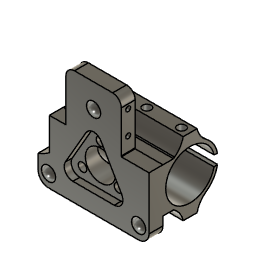
vacuum_pump_holder v3 (Autodesk Fusion 360 design; units mm, degrees)
Autodesk Fusion 360 part; units mm, degrees
sketch "Sketch1" plane through (0, 0, 0) normal (0, 1, 0) x (1, 0, 0)
  line L0 (-10.392305, 11.9) -> (10.392305, 11.9)
  arc A0 (-4.330127, -16.3) -> (4.330127, -16.3) centre (0, -13.8) ccw
  circle A1 centre (-25.980762, 15) radius 4.4
  circle A2 centre (0, -12) radius 2.475
  line L1 (0, 22.203919) -> (-7.3, 22.203919)
  line L2 (-16, -39.796081) -> (-16, -14.796081)
  line L3 (-11.951151, 11.9) -> (-10.392305, 11.9)
  line L4 (-32, 22.203919) -> (0, 22.203919)
  line L5 (32, 22.203919) -> (0, 22.203919)
  line L6 (5.10955, -14.95) -> (15.501855, 3.05)
  line L7 (-5.10955, -14.95) -> (-15.501855, 3.05)
  line L8 (0, -39.796081) -> (-16, -39.796081)
  line L9 (-32, -39.796081) -> (-32, 22.203919)
  arc A3 (-16, -14.796081) -> (-32, 7.874185) centre (-40.060655, -14.796081) ccw
  arc A4 (16.281278, 4.4) -> (11.951151, 11.9) centre (11.951151, 6.9) ccw
  circle A5 centre (0, 0) radius 8.75
  circle A6 centre (10.392305, 6) radius 2.475
  circle A7 centre (-10.392305, 6) radius 2.475
  line L10 (32, -39.796081) -> (32, 22.203919)
  line L11 (5.10955, -14.95) -> (4.330127, -16.3)
  line L12 (16, -39.796081) -> (16, -14.796081)
  line L13 (15.501855, 3.05) -> (16.281278, 4.4)
  arc A8 (32, 7.874185) -> (16, -14.796081) centre (40.060655, -14.796081) ccw
  line L14 (0, -39.796081) -> (16, -39.796081)
  arc A9 (-11.951151, 11.9) -> (-16.281278, 4.4) centre (-11.951151, 6.9) ccw
  circle A10 centre (25.980762, 15) radius 4.4
  line L15 (11.951151, 11.9) -> (10.392305, 11.9)
  line L16 (-5.10955, -14.95) -> (-4.330127, -16.3)
  line L17 (-15.501855, 3.05) -> (-16.281278, 4.4)
  circle A11 centre (0, -30) radius 1.6
  line L18 (-32, -39.796081) -> (-16, -39.796081)
  line L19 (16, -39.796081) -> (32, -39.796081)
  line L20 (-32, 22.203919) -> (-32, -1.546081)
  line L21 (-32, -1.546081) -> (-32, -13.796081)
  line L22 (32, 22.203919) -> (32, -1.546081)
  line L23 (32, -1.546081) -> (32, -15.546081)
  line L24 (0, 22.203919) -> (-12, 22.203919)
  line L25 (0, 22.203919) -> (12, 22.203919)
  line L26 (-12, 22.203919) -> (-12, 17.203919)
  circle A12 centre (12, 16.203919) radius 1.45
  circle A13 centre (12, -28.796081) radius 1.45
  line L27 (32, -39.796081) -> (32, -25.296081)
  arc A14 (32, -25.296081) -> (16, -39.796081) centre (30.570312, -39.796081) ccw
  line L28 (0, 0) -> (0, 22.203919)
  arc A15 (-16, -39.796081) -> (-32, -25.296081) centre (-30.570312, -39.796081) ccw
  circle A16 centre (-12, 16.203919) radius 1.45
  circle A17 centre (-12, -28.796081) radius 1.45
  line L29 (-32, -39.796081) -> (-32, -14.326081)
  arc A18 (-16, -39.796081) -> (-32, -14.326081) centre (-40.951887, -37.710087) ccw
  line L30 (-32, -14.326081) -> (-25.5, -14.326081)
  line L31 (-25.5, -14.326081) -> (-25.5, 4.358617)
  arc A19 (32, -14.326081) -> (16, -39.796081) centre (40.951887, -37.710087) ccw
  line L32 (-32, -14.326081) -> (-16.004591, -14.326081)
  line L33 (32, -14.326081) -> (16.004591, -14.326081)
  circle A20 centre (-25.980762, 15) radius 2.8
  circle A21 centre (25.980762, 15) radius 2.8
  circle A22 centre (0, -30) radius 2.8
  circle A23 centre (25.980762, 15) radius 1.75
  point P0 (-25.980762, 15)
  point P1 (25.980762, 15)
  dimension "d1" = 17.5
  dimension "d2" = 12
  dimension "d3" = 4.95
  dimension "d4" = 4.95
  dimension "d5" = 4.95
  dimension "d6" = 5.9
  dimension "d7" = 5.9
  dimension "d8" = 5
  dimension "d9" = 3.2
  dimension "d10" = 8.8
  dimension "d11" = 8.8
  dimension "d12" = 16
  dimension "d13" = 16
  dimension "d14" = 62
  dimension "d15" = 25
  dimension "d78" = 23.75
  dimension "d80" = 23.75
  dimension "d81" = 14
  dimension "d90" = 12
  dimension "d91" = 12
  dimension "d96" = 5
  dimension "d97" = 6
  dimension "d99" = 2.9
  dimension "d136" = 45
  dimension "d137" = 2.9
  dimension "d141" = 14.5
  dimension "d218" = 25.47
  dimension "d219" = 6.5
  dimension "d234" = 5.6
  dimension "d235" = 5.6
  dimension "d236" = 5.6
  dimension "d239" = 3.5
  constraint tangent A0 L11
  constraint tangent A0 L16
  constraint tangent A4 L13
  constraint tangent A4 L15
  constraint equal A0 A4
  constraint tangent L3 A9
  constraint tangent A9 L17
  constraint equal A0 A9
  constraint perpendicular L5 L10
  constraint tangent L12 A8
  constraint parallel L1 L4
  constraint perpendicular L2 L18
  constraint perpendicular L10 L19
  constraint perpendicular L4 L20
  constraint parallel L9 L21
  constraint perpendicular L5 L22
  constraint parallel L10 L23
  constraint parallel L4 L24
  constraint parallel L5 L25
  constraint perpendicular L4 L26
  constraint perpendicular L19 L27
  constraint tangent L12 A14
  constraint coincident A5.centre L28.start
  constraint perpendicular L4 L28
  constraint symmetric A14 L28 A15
  constraint symmetric A12 L28 A16
  constraint symmetric A13 L28 A17
  constraint perpendicular L18 L29
  constraint perpendicular L9 L30
  constraint perpendicular L30 L31
  constraint symmetric L28 A18 A19
  constraint perpendicular L2 L32
  constraint concentric A1 A20
  constraint concentric A10 A21
  constraint concentric A11 A22
  measures "d1" diameter of A5
  measures "d3" diameter of A2
  measures "d4" diameter of A6
  measures "d5" diameter of A7
  measures "d8" radius of A0
  measures "d9" diameter of A11
  measures "d10" diameter of A1
  measures "d11" diameter of A10
  measures "d99" diameter of A12
  measures "d137" diameter of A13
  measures "d234" diameter of A20
  measures "d235" diameter of A21
  measures "d236" diameter of A22
  measures "d239" diameter of A23
sketch "bottom" plane through (0, 0, 39.796081) normal (0, 0, 1) x (-1, 0, 0)
  line L0 (32, 0) -> (-32, 0)
  line L1 (-32, 0) -> (-32, -10)
  line L2 (-32, -10) -> (32, -10)
  line L3 (32, -10) -> (32, 0)
  line L4 (32, 0) -> (32, -19.73)
  line L5 (-32, 0) -> (-32, -19.73)
  line L6 (0, 0) -> (0, -19.73)
  circle A0 centre (0, -19.73) radius 14
  circle A1 centre (0, -19.73) radius 12.25
  line L7 (0, -19.73) -> (21.8, -19.73)
  line L8 (21.8, -19.73) -> (21.8, -22.73)
  line L9 (21.8, -19.73) -> (21.8, -16.73)
  line L10 (21.8, -16.73) -> (13.674794, -16.73)
  line L11 (21.8, -22.73) -> (13.674794, -22.73)
  line L12 (0, -30) -> (12, -30)
  line L13 (0, -30) -> (-12, -30)
  arc A2 (-12, -30) -> (12, -30) centre (0, -20.125001) ccw
  line L14 (32, -19.73) -> (12, -30)
  line L15 (-12, -30) -> (-32, -19.73)
  dimension "d22" = 19.73
  dimension "d23" = 19.73
  dimension "d29" = 19.73
  dimension "d30" = 28
  dimension "d31" = 24.5
  dimension "d32" = 21.8
  dimension "d33" = 3
  dimension "d34" = 3
  dimension "d35" = 12
  constraint coincident L0.start L3.end
  constraint perpendicular L0 L4
  constraint coincident L0.end L1.start
  constraint perpendicular L0 L5
  constraint coincident L6.start origin
  constraint perpendicular L0 L6
  constraint coincident L6.end A0.centre
  constraint concentric A0 A1
  constraint perpendicular L6 L7
  constraint perpendicular L7 L8
  constraint perpendicular L7 L9
  constraint perpendicular L9 L10
  constraint perpendicular L8 L11
  constraint horizontal L12
  constraint parallel L12 L13
  measures "d22" distance of L0.start L4.end
  measures "d23" distance of L0.end L5.end
  measures "d29" distance of L6.start L6.end
  measures "d30" diameter of A0
  measures "d31" diameter of A1
  measures "d32" distance of L6.end L7.end
  measures "d33" distance of L7.end L8.end
  measures "d34" distance of L7.end L9.end
  measures "d35" distance of L12.start L13.end
extrude "Extrude4" add sketch "Sketch1" along normal blind 39.46 contours L0 A0 L3 L6 L7 A4 L11 L13 A9 L15 L16 L17 | A1 | A2 | L1 L2 L4 L5 L8 L9 A3 L10 L12 A8 L14 L20 L22 L24 L25 A18 A19 | L10 A8 L22 L23 L33 | L9 A3 L20 L21 L30 L31 L32 | L12 A8 A19 L33 | A3 L31 L32 | L10 L12 L23 A14 A19 | L2 A3 A18 L30 L32 | L12 A19 | L2 L9 A15 L29 A18 | L10 L19 L27 A14 | L9 L18 A15 L29 | L2 A18 | A5 | A6 | A7 | A10 | A11 | A12 | A13 | A16 | A17 | A20 | A21 | A22 | A23 picked at (-4.711137, 10.569969) picked at (-22.140901, 14.642299) picked at (-0.18358, -11.195684) picked at (-10.740589, -19.482072) picked at (27.37273, -6.932301) picked at (-27.666667, -3.837848) picked at (20.054611, -19.162446) picked at (-19.256218, -13.297778) picked at (28.224316, -19.587338) picked at (-21.577044, -16.380874) picked at (15.974211, -37.478071) picked at (-30.939878, -18.476301) picked at (21.380237, -39.122729) picked at (-21.380237, -39.122729) picked at (-15.974211, -37.942103) picked at (-0.424451, 2.741984) picked at (10.956125, 6.501084) picked at (-10.123158, 6.626633) picked at (29.820623, 14.642299) picked at (-0.142372, -29.637241) picked at (12.435468, 15.994209) picked at (12.46186, -28.938546) picked at (-11.895495, 15.822215) picked at (-11.53814, -28.938546) picked at (-25.639777, 14.04895) picked at (28.413822, 14.773953) picked at (2.383619, -30.218595) picked at (27.031686, 14.71542)
sketch "side2" plane through (32, 0, 0) normal (1, 0, 0) x (0, 1, 0)
  line L0 (0, 39.796081) -> (0, -22.203919)
  line L1 (0, -22.203919) -> (39.46, -22.203919)
  line L2 (39.46, -22.203919) -> (39.46, 39.796081)
  line L3 (39.46, 39.796081) -> (0, 39.796081)
  line L4 (19.73, -22.203919) -> (5.73, -22.203919)
  circle A0 centre (19.73, 1.546081) radius 14.1
  circle A1 centre (19.73, 1.546081) radius 16
  line L5 (19.73, 1.546081) -> (19.73, 4.546081)
  line L6 (19.73, 4.546081) -> (43.73, 4.546081)
  line L7 (43.73, 4.546081) -> (43.73, -1.453919)
  line L8 (43.73, -1.453919) -> (35.446234, -1.453919)
  line L9 (19.73, 1.546081) -> (43.73, 1.546081)
  line L10 (0, -22.203919) -> (4, -22.203919)
  line L11 (4, -22.203919) -> (4, 39.796081)
  line L12 (4, -22.203919) -> (4, -17.203919)
  line L13 (39.46, 1.546081) -> (39.46, -4.453919)
  line L14 (39.46, 1.546081) -> (39.46, 7.546081)
  line L15 (43.73, 4.546081) -> (39.46, 7.546081)
  line L16 (39.46, 7.546081) -> (29.357219, 14.325621)
  line L17 (39.46, -4.453919) -> (29.357219, -11.23346)
  line L18 (43.73, -1.453919) -> (39.46, -4.453919)
  line L19 (39.46, 25.296081) -> (4, 25.296081)
  line L20 (29.357219, 14.325621) -> (29.357219, 25.296081)
  line L21 (29.357219, -11.23346) -> (29.357219, -22.203919)
  line L22 (19.73, 17.546081) -> (19.73, 22.546081)
  line L23 (19.73, 22.546081) -> (29.357219, 22.546081)
  line L24 (19.73, 22.546081) -> (23.73, 22.546081)
  line L25 (19.73, 22.546081) -> (4, 22.546081)
  arc A2 (23.73, 22.546081) -> (29.357219, 14.325621) centre (36.849635, 25.49072) ccw
  arc A3 (4, 25.296081) -> (19.73, 22.546081) centre (20.714595, 74.540765) ccw
  line L26 (19.73, -19.453919) -> (23.73, -19.453919)
  arc A4 (29.357219, -11.23346) -> (23.73, -19.453919) centre (36.849635, -22.398558) ccw
  arc A5 (19.73, -19.453919) -> (4, -22.203919) centre (20.714595, -71.448604) ccw
  arc A6 (10.102781, 14.325621) -> (15.73, 22.546081) centre (2.610365, 25.49072) ccw
  arc A7 (4, 22.546081) -> (10.102781, 14.325621) centre (41.738131, 44.186915) ccw
  arc A8 (15.73, -19.453919) -> (10.102781, -11.23346) centre (2.610365, -22.398558) ccw
  line L27 (15.73, -19.453919) -> (23.73, -19.453919)
  line L28 (10.102781, 14.325621) -> (4, 14.325621)
  line L29 (10.102781, -11.23346) -> (4, -11.23346)
  line L30 (35.446234, -1.453919) -> (33.507155, -1.453919)
  line L31 (33.507155, 4.546081) -> (40.904794, 4.546081)
  line L32 (40.904794, 1.546081) -> (40.904794, -0.953919)
  line L33 (40.904794, 1.546081) -> (40.904794, 4.046081)
  arc A9 (33.507155, 4.546081) -> (40.904794, 4.046081) centre (40.110525, 47.269716) ccw
  arc A10 (40.904794, -0.953919) -> (33.507155, -1.453919) centre (40.110525, -44.177555) ccw
  line L34 (0, 39.796081) -> (-4, 39.796081)
  dimension "d50" = 19.73
  dimension "d53" = 14
  dimension "d60" = 28.2
  dimension "d102" = 32
  dimension "d105" = 3
  dimension "d107" = 24
  dimension "d108" = 6
  dimension "d114" = 4
  dimension "d115" = 5
  dimension "d118" = 6
  dimension "d119" = 6
  dimension "d165" = 5
  dimension "d166" = 4
  dimension "d171" = 2.5
  dimension "d172" = 2.5
  dimension "d251" = 4
  constraint concentric A0 A1
  constraint vertical L5
  constraint perpendicular L2 L6
  constraint perpendicular L6 L7
  constraint perpendicular L5 L8
  constraint perpendicular L0 L10
  constraint perpendicular L3 L11
  constraint perpendicular L10 L12
  constraint perpendicular L8 L13
  constraint perpendicular L6 L14
  constraint perpendicular L11 L19
  constraint perpendicular L19 L20
  constraint perpendicular L1 L21
  constraint perpendicular L19 L22
  constraint perpendicular L20 L23
  constraint perpendicular L22 L24
  constraint perpendicular L11 L25
  constraint tangent L16 A2
  constraint symmetric L9 A2 A4
  constraint symmetric L9 A3 A5
  constraint symmetric L22 A2 A6
  constraint symmetric L9 A6 A8
  constraint perpendicular L11 L28
  constraint perpendicular L11 L29
  constraint parallel L8 L30
  constraint perpendicular L14 L31
  constraint perpendicular L9 L32
  constraint perpendicular L9 L33
  constraint symmetric L9 A9 A10
  constraint perpendicular L0 L34
  measures "d60" diameter of A0
  measures "d102" diameter of A1
sketch "top" plane through (0, 39.46, 0) normal (0, 1, 0) x (-1, 0, 0)
  line L0 (32, 39.796081) -> (-32, 39.796081)
  line L1 (-32, 39.796081) -> (-32, -22.203919)
  line L2 (-32, -22.203919) -> (32, -22.203919)
  line L3 (32, -22.203919) -> (32, 39.796081)
  line L4 (-32, -22.203919) -> (-32, -12.203919)
  line L5 (-32, -12.203919) -> (-4.5, -12.203919)
  line L6 (-4.5, -12.203919) -> (-4.5, 15.796081)
  line L7 (-4.5, 15.796081) -> (-32, 15.796081)
  line L8 (-4.5, -12.203919) -> (-4.5, 1.796081)
  line L9 (-32, -12.203919) -> (-32, 1.796081)
  line L10 (-32, 1.796081) -> (-13.1, 1.796081)
  circle A0 centre (-13.1, 1.796081) radius 3
  line L11 (-32, 1.796081) -> (25.5, 1.796081)
  line L12 (25.5, 1.796081) -> (25.5, 14.046081)
  line L13 (25.5, 14.046081) -> (-4.5, 14.046081)
  line L14 (25.5, -10.453919) -> (-4.5, -10.453919)
  line L15 (25.5, 1.796081) -> (25.5, -10.453919)
  line L16 (32, 39.796081) -> (-32, 39.796081)
  line L17 (0, -22.203919) -> (-12, -22.203919)
  line L18 (0, -22.203919) -> (12, -22.203919)
  line L19 (-12, -22.203919) -> (-12, -16.203919)
  circle A1 centre (-12, -16.203919) radius 2.75
  line L20 (12, -22.203919) -> (12, -16.203919)
  circle A2 centre (12, -16.203919) radius 2.75
  circle A3 centre (-12, 28.796081) radius 2.75
  line L21 (0, 39.796081) -> (0, -22.203919)
  circle A4 centre (12, 28.796081) radius 2.75
  dimension "d61" = 10
  dimension "d62" = 27.5
  dimension "d63" = 28
  dimension "d64" = 14
  dimension "d65" = 18.9
  dimension "d66" = 6
  dimension "d67" = 57.5
  dimension "d68" = 12.25
  dimension "d126" = 12
  dimension "d127" = 12
  dimension "d128" = 6
  dimension "d129" = 5.5
  dimension "d130" = 6
  dimension "d131" = 5.5
  dimension "d139" = 45
  dimension "d140" = 5.5
  constraint perpendicular L2 L4
  constraint perpendicular L4 L5
  constraint perpendicular L5 L6
  constraint perpendicular L1 L7
  constraint perpendicular L5 L9
  constraint perpendicular L9 L10
  constraint perpendicular L9 L11
  constraint perpendicular L11 L12
  constraint perpendicular L6 L13
  constraint parallel L2 L17
  constraint parallel L2 L18
  constraint perpendicular L17 L19
  constraint perpendicular L18 L20
  constraint symmetric A3 L21 A4
  measures "d66" diameter of A0
  measures "d129" diameter of A1
  measures "d131" diameter of A2
  measures "d140" diameter of A3
sketch "side1" plane through (-32, 0, 0) normal (-1, 0, 0) x (0, -1, 0)
  line L0 (0, -22.203919) -> (0, 39.796081)
  line L1 (0, 39.796081) -> (-39.46, 39.796081)
  line L2 (-39.46, 39.796081) -> (-39.46, -22.203919)
  line L3 (-39.46, -22.203919) -> (0, -22.203919)
  line L4 (0, -22.203919) -> (-19.73, -22.203919)
  line L5 (-19.73, -22.203919) -> (-19.73, 1.546081)
  circle A0 centre (-19.73, 1.546081) radius 12.65
  line L6 (0, -22.203919) -> (-4, -22.203919)
  line L7 (-4, -22.203919) -> (-4, 39.796081)
  line L8 (-41.73, 4.546081) -> (-41.73, -1.453919)
  circle A1 centre (-19.73, 1.546081) radius 14.25
  line L9 (-4, -22.203919) -> (-4, -17.203919)
  arc A2 (-41.73, 4.546081) -> (-29.866601, 11.56166) centre (-49.126004, 30.591122) ccw
  arc A3 (-29.866601, -8.469498) -> (-41.73, -1.453919) centre (-49.126004, -27.498961) ccw
  arc A4 (-4, -22.203919) -> (-19.73, -12.703919) centre (-19.496567, -30.090188) ccw
  arc A5 (-19.73, 15.796081) -> (-4, 25.296081) centre (-19.496567, 33.18235) ccw
  circle A6 centre (-19.73, 1.546081) radius 3.25
  circle A7 centre (-19.73, 1.546081) radius 10
  circle A8 centre (-19.73, 1.546081) radius 8.15
  circle A9 centre (-19.73, 1.546081) radius 13
  circle A10 centre (-19.73, 1.546081) radius 7
  line L10 (-19.73, 4.796081) -> (-31.955383, 4.796081)
  line L11 (-19.73, -1.703919) -> (-31.955383, -1.703919)
  line L12 (-19.73, 4.796081) -> (-7.504617, 4.796081)
  line L13 (-19.73, -1.703919) -> (-7.504617, -1.703919)
  dimension "d71" = 19.73
  dimension "d72" = 23.75
  dimension "d73" = 25.3
  dimension "d82" = 4
  dimension "d111" = 6
  dimension "d112" = 28.5
  dimension "d113" = 5
  dimension "d179" = 6.5
  dimension "d180" = 20
  dimension "d181" = 16.3
  dimension "d182" = 26
  dimension "d190" = 14
  constraint perpendicular L0 L4
  constraint perpendicular L4 L5
  constraint perpendicular L0 L6
  constraint perpendicular L1 L7
  constraint concentric A0 A1
  constraint perpendicular L4 L9
  constraint tangent A1 A2
  constraint concentric A0 A6
  constraint concentric A1 A7
  constraint concentric A6 A8
  constraint concentric A7 A9
  constraint concentric A8 A10
  constraint tangent A6 L10
  constraint horizontal L10
  constraint tangent A6 L11
  constraint parallel L11 L12
  constraint parallel L12 L13
  measures "d73" diameter of A0
  measures "d112" diameter of A1
  measures "d179" diameter of A6
  measures "d180" diameter of A7
  measures "d181" diameter of A8
  measures "d182" diameter of A9
  measures "d190" diameter of A10
sketch "high" plane through (0, 0, 39.796081) normal (0, 0, 1) x (-1, 0, 0)
  line L0 (32, 0) -> (-32, 0)
  line L1 (-32, 0) -> (-32, -39.46)
  line L2 (-32, -39.46) -> (32, -39.46)
  line L3 (32, -39.46) -> (32, 0)
  line L4 (-32, 0) -> (-32, -19.73)
  line L5 (-32, -19.73) -> (-27, -19.73)
  circle A0 centre (-27, -19.73) radius 2.45
  line L6 (-4.5, -5.73) -> (-32, -5.73)
  line L7 (-4.5, -33.73) -> (-4.5, -5.73)
  line L8 (-32, -33.73) -> (-4.5, -33.73)
  line L9 (25.5, -31.98) -> (-4.5, -31.98)
  line L10 (25.5, -19.73) -> (25.5, -31.98)
  line L11 (25.5, -19.73) -> (25.5, -7.48)
  line L12 (25.5, -7.48) -> (-4.5, -7.48)
  line L13 (-32, -39.46) -> (25.5, -39.46)
  circle A1 centre (-7, -19.73) radius 2.45
  circle A2 centre (7, -19.73) radius 2.45
  line L14 (16, -19.73) -> (7, -19.73)
  line L15 (16, -19.73) -> (7, -19.73)
  line L16 (16, -19.73) -> (-16, -19.73)
  point P0 (-32, -19.73)
  point P1 (25.5, -19.73)
  point P2 (-7, -19.73)
  point P3 (7, -19.73)
  dimension "d158" = 5
  dimension "d159" = 4.9
  dimension "d199" = 27.5
  dimension "d200" = 28
  dimension "d201" = 12.25
  dimension "d202" = 57.5
  dimension "d203" = 19.73
  dimension "d215" = 4.9
  dimension "d217" = 4.9
  dimension "d244" = 9
  constraint coincident L0.end L1.start
  constraint midpoint L1 P0
  constraint perpendicular L4 L5
  constraint coincident L5.end A0.centre
  constraint perpendicular L7 L8
  constraint coincident L12.end L7
  constraint perpendicular L7 L12
  constraint coincident L1.end L2.start
  constraint perpendicular L1 L13
  constraint coincident P0 L4.end
  constraint parallel L14 L15
  constraint coincident P3 A2.centre
  constraint parallel L14 L16
  measures "d158" distance of P0 L5.end
  measures "d159" diameter of A0
  measures "d199" distance of L7.start L8.start
  measures "d200" distance of L7.start L6.start
  measures "d201" distance of L11.end P1
  measures "d202" distance of L1.end L13.end
  measures "d203" distance of L13.end P1
  measures "d215" diameter of A1
  measures "d217" diameter of A2
  measures "d244" distance of L14.start P3
sketch "low" plane through (0, 0, -22.203919) normal (0, 0, -1) x (1, 0, 0)
  line L0 (32, 0) -> (-32, 0)
  line L1 (-32, 0) -> (-32, -39.46)
  line L2 (-32, -39.46) -> (32, -39.46)
  line L3 (32, -39.46) -> (32, 0)
  line L4 (32, -39.46) -> (32, -19.73)
  line L5 (32, -19.73) -> (27, -19.73)
  circle A0 centre (27, -19.73) radius 1.425
  line L6 (32, -19.73) -> (12, -19.73)
  line L7 (32, -19.73) -> (0, -19.73)
  line L8 (12, -19.73) -> (-12, -19.73)
  circle A1 centre (12, -19.73) radius 2.75
  circle A2 centre (-12, -19.73) radius 2.75
  line L9 (-12, -19.73) -> (-5, -19.73)
  circle A3 centre (0, -19.73) radius 2.45
  line L10 (32, -19.73) -> (19, -19.73)
  dimension "d160" = 2.85
  dimension "d204" = 20
  dimension "d205" = 32
  dimension "d206" = 24
  dimension "d207" = 5.5
  dimension "d208" = 5.5
  dimension "d209" = 7
  dimension "d211" = 4.9
  dimension "d252" = 13
  constraint coincident L2.end L3.start
  constraint midpoint L3 L4.end
  constraint perpendicular L4 L5
  constraint coincident L5.end A0.centre
  constraint perpendicular L4 L6
  constraint coincident L6 L7.end
  constraint parallel L6 L8
  constraint coincident L6.end L8.start
  constraint coincident L8.end A2.centre
  constraint parallel L8 L9
  constraint coincident L7.end A3.centre
  constraint perpendicular L4 L10
  measures "d160" diameter of A0
  measures "d204" distance of L4.end L6.end
  measures "d205" distance of L4.end L7.end
  measures "d206" distance of L6.end L8.end
  measures "d207" diameter of A1
  measures "d208" diameter of A2
  measures "d209" distance of L8.end L9.end
  measures "d211" diameter of A3
  measures "d252" distance of L4.end L10.end
extrude "Extrude14" add sketch "side2" against normal blind 57.5 contours L2 L6 L14 L15 L31 | L2 L6 L7 L9 L14 L31 L33 A9 | L2 L9 L14 L33 A9 | L2 L7 L8 L9 L13 L32 A10 | L2 L8 L13 L18 | L2 L9 L13 L32 A10 picked at (41.364931, 5.546081) picked at (42.788265, 3.379414) picked at (40.10213, 2.377092) picked at (42.788265, -0.287253) picked at (40.883333, -2.453919) picked at (40.10213, 0.71507)
sketch "Sketch12" plane through (0, 43.73, 0) normal (0, 1, 0) x (-1, 0, 0)
  line L0 (-32, 4.546081) -> (-32, -1.453919)
  line L1 (-32, -1.453919) -> (25.5, -1.453919)
  line L2 (25.5, -1.453919) -> (25.5, 4.546081)
  line L3 (25.5, 4.546081) -> (-32, 4.546081)
  circle A0 centre (-10.89, 1.796081) radius 3.65
  line L4 (-38.5, 1.796081) -> (19, 1.796081)
  line L5 (19, 1.796081) -> (25.5, 1.796081)
  line L6 (19, 1.796081) -> (19, 25.546081)
  line L7 (19, 25.546081) -> (25.5, 25.546081)
  line L8 (-10.89, 1.796081) -> (-32, 1.796081)
  dimension "d150" = 7.3
  dimension "d151" = 57.5
  dimension "d176" = 23.75
  constraint perpendicular L2 L5
  constraint perpendicular L3 L6
  constraint perpendicular L6 L7
  constraint perpendicular L0 L8
  measures "d150" diameter of A0
extrude "Extrude5" cut sketch "side2" against normal blind 27.5 contours A0 L5 L6 L9 | A0 L5 L6 L9 picked at (15.08025, 3.231517) picked at (24.322385, 3.546081)
extrude "Extrude16" cut sketch "Sketch12" against normal blind 13 contours L3 A0 | L3 A0 L4 L8 | L1 A0 L4 L8 | L1 A0 picked at (-10.715997, 4.833574) picked at (-10.89, 3.629414) picked at (-10.89, -0.370586) picked at (-11.292914, -1.518601)
sketch "Sketch13" plane through (0, 16.590422, 23.6137) normal (0, 0.574876, 0.81824) x (-1, 0, 0)
  ellipse E0 centre (-10.89, -37.951859) end of major axis (-10.89, -44.301052) minor radius 3.65 (-8.49, -33.16822) -> (-13.29, -33.16822) ccw
  line L0 (-8.49, -33.16822) -> (25.5, -33.16822)
  line L1 (25.5, -33.16822) -> (25.5, -27.949705)
  line L2 (-32, -27.949705) -> (-32, -33.16822)
  line L3 (-32, -33.16822) -> (-13.29, -33.16822)
  line L4 (-32, -27.949705) -> (-5, -27.949705)
  line L5 (25.5, -27.949705) -> (-32, -27.949705)
  dimension "d154" = 27
  constraint perpendicular L2 L4
extrude "Extrude10" cut sketch "side1" against normal blind 36.5 contours L1 L2 L7 A1 A2 A5 | L2 L3 L5 A1 A3 picked at (-21.063333, 31.796081) picked at (-28.137582, -18.670203)
extrude "Extrude13" cut sketch "Sketch1" along normal blind 4 contours L10 L19 L27 A14 | L9 L18 A15 L29 picked at (21.380237, -39.122729) picked at (-21.380237, -39.122729)
extrude "Extrude11" cut sketch "side1" against normal blind 36.5 contours L3 L4 L5 A4 picked at (-18.925216, -15.915836)
extrude "Extrude6" cut sketch "side1" against normal blind 36.5 contours L5 A0 A7 L11 | L5 A0 A7 L13 | L5 A7 A8 L11 | L5 A7 A8 L13 | A0 A7 L10 L11 | A0 A7 L12 L13 | L5 A8 A10 L11 | L5 A8 A10 L13 | A7 A8 L10 L11 | A7 A8 L12 L13 | A0 A7 L10 L12 | L5 A10 L11 | L5 A10 L13 | A8 A10 L10 L11 | A8 A10 L12 L13 | A7 A8 L10 L12 | A6 A10 L10 L11 | A6 | A6 A10 L12 L13 | A8 A10 L10 L12 | A10 L10 L12 picked at (-30.832236, -2.283944) picked at (-8.627764, -2.283944) picked at (-28.347454, -2.126537) picked at (-11.112546, -2.126537) picked at (-31.45383, 0.779297) picked at (-9.010873, 3.369518) picked at (-26.596448, -2.052706) picked at (-12.863552, -2.052706) picked at (-29.098729, 1.546081) picked at (-11.470575, 4.446402) picked at (-20.584922, 13.259232) picked at (-20.046347, -4.182375) picked at (-19.413653, -4.182375) picked at (-27.465765, 2.077179) picked at (-12.440944, 4.189672) picked at (-19.73, 10.911693) picked at (-25.000986, 3.814056) picked at (-19.004433, 0.640462) picked at (-14.495955, -0.813889) picked at (-20.291837, 9.278073) picked at (-19.73, 7.283811)
extrude "Extrude9" cut sketch "side2" against normal blind 27.5 contours L2 L3 L11 L19 | L1 L4 A1 L21 L26 A4 A5 L27 | L19 L20 L23 L24 A3 | L2 L16 L19 L20 | A1 L20 L23 A2 | L1 L2 L17 L21 picked at (24.272406, 34.962747) picked at (24.272406, -21.287253) picked at (27.481479, 23.462747) picked at (36.092406, 15.722594) picked at (26.226645, 20.775954) picked at (36.092406, -12.630433)
extrude "Extrude15" add 2 faces at (4.5, 17.149068, 20.466426) (4.5, 17.149068, -17.374265) along direction (-1, 0, 0) blind 30
extrude "Extrude19" cut sketch "side2" against normal blind 64 contours A1 L11 L12 A5 A8 L27 L29 | L11 L25 A3 | L11 A7 L28 | A1 L25 A6 A7 picked at (8.434766, -16.963491) picked at (5.713239, 23.894477) picked at (5.890472, 16.959028) picked at (8.515493, 21.580266)
extrude "Extrude20" cut sketch "side2" against normal blind 27 contours L2 L9 L14 L33 A9 | L2 A1 L9 L14 A9 | L2 L9 L13 L32 A10 | L2 A1 L9 L13 A10 | A0 A1 L9 A9 | A0 A1 L9 A10 picked at (40.10213, 2.377092) picked at (37.766432, 2.697804) picked at (40.10213, 0.71507) picked at (37.766432, 0.394357) picked at (34.368342, 3.161763) picked at (34.368342, -0.069601)
sketch "Sketch17" plane through (-32, 0, 0) normal (-1, 0, 0) x (0, -1, 0)
  circle A0 centre (-19.73, 1.546081) radius 12.65
  line L0 (-4, 25.296081) -> (-4, 14.325621)
  line L1 (-4, 14.325621) -> (-10.102781, 14.325621)
  arc A1 (-10.102781, 14.325621) -> (-10.751632, 14.789529) centre (-19.73, 1.546081) ccw
  arc A2 (-13.060446, 17.029542) -> (-10.751632, 14.789529) centre (-2.610365, 25.49072) ccw
  arc A3 (-19.51972, 15.794529) -> (-13.060446, 17.029542) centre (-19.496567, 33.18235) ccw
  arc A4 (-19.51972, 15.794529) -> (-29.866601, 11.56166) centre (-19.73, 1.546081) ccw
  arc A5 (-39.46, 5.300542) -> (-29.866601, 11.56166) centre (-49.126004, 30.591122) ccw
  line L2 (-39.46, 5.300542) -> (-39.46, -2.208381)
  arc A6 (-29.866601, -8.469498) -> (-39.46, -2.208381) centre (-49.126004, -27.498961) ccw
  arc A7 (-29.866601, -8.469498) -> (-19.51972, -12.702368) centre (-19.73, 1.546081) ccw
  arc A8 (-13.060446, -13.937381) -> (-19.51972, -12.702368) centre (-19.496567, -30.090188) ccw
  arc A9 (-10.751632, -11.697367) -> (-13.060446, -13.937381) centre (-2.610365, -22.398558) ccw
  arc A10 (-10.751632, -11.697367) -> (-10.102781, -11.23346) centre (-19.73, 1.546081) ccw
  line L3 (-10.102781, -11.23346) -> (-4, -11.23346)
  line L4 (-4, -11.23346) -> (-4, -22.203919)
  line L5 (-4, -22.203919) -> (0, -22.203919)
  line L6 (0, -22.203919) -> (0, 25.296081)
  line L7 (0, 25.296081) -> (-4, 25.296081)
  line L8 (-4, 14.325621) -> (-4, -11.23346)
extrude "Extrude21" cut sketch "Sketch17" against normal blind 6.5 contours L1 A1 A2 A3 A4 A5 L2 A6 A7 A8 A9 A10 L3 L8 picked at (-37.1, 1.546081)
extrude "Extrude22" add sketch "side1" against normal blind 6.5 draft 20 from surface at -4.5 contours A1 A4 A5 | L5 A0 A7 L11 | L5 A0 A7 L13 | A0 A7 L10 L11 | A0 A7 L12 L13 | A0 A7 L10 L12 | A9 picked at (-27.957999, -9.021653) picked at (-30.832236, -2.283944) picked at (-8.627764, -2.283944) picked at (-31.45383, 0.779297) picked at (-9.010873, -0.277356) picked at (-20.584922, 13.259232) picked at (-31.75988, 5.752629)
extrude "Extrude24" cut 1 faces at (-21, 8.827455, 0.538347) along direction (-1, 0, 0) blind 7
extrude "Extrude27" add sketch "side1" against normal blind 2 from surface at -4.5 contours A0 A7 L10 L11 | A0 A7 L12 L13 | A7 A8 L10 L11 | A7 A8 L12 L13 | L5 A10 L11 | L5 A10 L13 | A8 A10 L10 L11 | A8 A10 L12 L13 | A6 A10 L10 L11 | A6 A10 L12 L13 | A10 L10 L12 picked at (-31.45383, 0.779297) picked at (-9.010873, 3.369518) picked at (-29.098729, 1.546081) picked at (-11.470575, 4.446402) picked at (-20.046347, -4.182375) picked at (-19.413653, -4.182375) picked at (-27.465765, 2.077179) picked at (-12.440944, 4.189672) picked at (-25.000986, 3.814056) picked at (-14.495955, -0.813889) picked at (-19.73, 7.283811)
extrude "Extrude17" cut sketch "low" against normal blind 7 contours L5 A0 L6 L7 L10 | L5 A0 L6 L7 L10 | L7 L8 A3 | L7 L8 A3 picked at (26.055306, -19.800795) picked at (26.355643, -19.035548) picked at (1.624212, -19.851718) picked at (-1.624212, -19.608282)
extrude "Extrude18" cut sketch "high" against normal blind 22.25 contours A0 | A1 L16 | A1 L16 | A2 L14 L15 L16 | A2 L14 L15 L16 picked at (-26.728149, -19.145674) picked at (-6.938971, -18.915617) picked at (-7.06103, -20.544383) picked at (8.107842, -18.53603) picked at (5.375788, -19.851718)
extrude "Extrude29" cut sketch "Sketch1" along normal blind 4 contours L9 A3 L20 L21 L30 L31 L32 | L12 A8 A19 L33 | L10 L12 L23 A14 A19 | L2 A3 A18 L30 L32 | L2 L9 A15 L29 A18 picked at (-27.666667, -3.837848) picked at (20.054611, -19.162446) picked at (28.224316, -19.587338) picked at (-21.577044, -16.380874) picked at (-30.939878, -18.476301)
extrude "Extrude30" cut 4 faces at (-21, 9.817899, -11.520015) (-21, 29.653545, -11.487824) (-21, 9.817899, 14.612177) (-21, 29.653545, 14.579985) along direction (-1, 0, 0) blind 2.5
extrude "Extrude32" cut sketch "Sketch1" against normal blind 20 from the near side of the face at (-6.333333, 23.881566, -18.845405) contours A23 picked at (27.031686, 14.71542)
extrude "Extrude35" cut sketch "side2" against normal blind 59 contours L2 L6 L14 L15 L31 | L2 A1 L6 L14 L16 L31 | L2 L6 L7 L9 L14 L31 L33 A9 | L2 A1 L6 L14 L31 A9 | L2 A1 L8 L13 L17 | L2 L9 L14 L33 A9 | L2 A1 L9 L14 A9 | L2 L7 L8 L9 L13 L32 A10 | L2 L8 L13 L18 | L2 A1 L8 L13 A10 | L2 L9 L13 L32 A10 | L2 A1 L9 L13 A10 picked at (41.364931, 5.546081) picked at (38.122078, 5.546081) picked at (42.788265, 3.379414) picked at (39.018538, 4.224559) picked at (38.122078, -2.453919) picked at (40.10213, 2.377092) picked at (37.766432, 2.697804) picked at (42.788265, -0.287253) picked at (40.883333, -2.453919) picked at (39.018538, -1.132397) picked at (40.10213, 0.71507) picked at (37.766432, 0.394357)
extrude "Extrude36" add sketch "Sketch1" against normal blind 4 contours A1 | L1 L2 L4 L5 L8 L9 A3 L10 L12 A8 L14 L20 L22 L24 L25 A18 A19 | A10 | A11 | A12 | A13 | A16 | A17 | A20 | A21 | A22 | A23 picked at (-22.140901, 14.642299) picked at (-10.740589, -19.482072) picked at (29.820623, 14.642299) picked at (-0.142372, -29.637241) picked at (12.435468, 15.994209) picked at (12.46186, -28.938546) picked at (-11.895495, 15.822215) picked at (-11.53814, -28.938546) picked at (-25.639777, 14.04895) picked at (28.413822, 14.773953) picked at (2.383619, -30.218595) picked at (27.031686, 14.71542)
extrude "Extrude37" cut sketch "Sketch1" along normal blind 4.2 contours A2 | A6 | A7 picked at (-0.18358, -11.195684) picked at (10.956125, 6.501084) picked at (-10.123158, 6.626633)
extrude "Extrude38" cut sketch "Sketch1" along normal blind 10 contours A5 picked at (-0.424451, 2.741984)
extrude "Extrude31" cut sketch "Sketch1" against normal blind 3 from surface at 4 contours A11 | A20 | A21 | A22 | A23 picked at (-0.142372, -29.637241) picked at (-25.639777, 14.04895) picked at (28.413822, 14.773953) picked at (2.383619, -30.218595) picked at (27.031686, 14.71542)
sphere "SpherePrimitive2" cut diameter 8.2 placed x (1, 0, 0) y (0, 0, 1) z (0, -1, 0) at (26, -4, -15)
sphere "SpherePrimitive3" cut diameter 8.2 placed x (1, 0, 0) y (0, 0, 1) z (0, -1, 0) at (-26, -4, -15)
sphere "SpherePrimitive4" cut diameter 8.2 placed x (1, 0, 0) y (0, 0, 1) z (0, -1, 0) at (0, -4, 30)
sketch "Sketch23" plane through (0, -4, 0) normal (0, -1, 0) x (1, 0, 0)
  circle A0 centre (0, 30) radius 4.1
  circle A1 centre (-26, -15) radius 4.1
  circle A2 centre (26, -15) radius 4.1
  line L0 (-16.281278, -4.4) -> (-4.330127, 16.3)
  arc A3 (4.330127, 16.3) -> (-4.330127, 16.3) centre (0, 13.8) ccw
  line L1 (4.330127, 16.3) -> (16.281278, -4.4)
  arc A4 (11.951151, -11.9) -> (16.281278, -4.4) centre (11.951151, -6.9) ccw
  line L2 (11.951151, -11.9) -> (-11.951151, -11.9)
  arc A5 (-16.281278, -4.4) -> (-11.951151, -11.9) centre (-11.951151, -6.9) ccw
  line L3 (-32, -22.203919) -> (32, -22.203919)
  line L4 (32, -22.203919) -> (32, -7.874185)
  arc A6 (16, 14.796081) -> (32, -7.874185) centre (40.060655, 14.796081) ccw
  line L5 (16, 14.796081) -> (16, 35.624093)
  arc A7 (16, 39.796081) -> (16, 35.624093) centre (40.951887, 37.710087) ccw
  line L6 (16, 39.796081) -> (-16, 39.796081)
  arc A8 (-16, 35.624093) -> (-16, 39.796081) centre (-40.951887, 37.710087) ccw
  line L7 (-16, 35.624093) -> (-16, 14.796081)
  arc A9 (-32, -7.874185) -> (-16, 14.796081) centre (-40.060655, 14.796081) ccw
  line L8 (-32, -7.874185) -> (-32, -22.203919)
  circle A10 centre (-26, -15) radius 1.45
  circle A11 centre (26, -15) radius 1.45
  circle A12 centre (0, 30) radius 1.45
  dimension "d266" = 2.9
  dimension "d267" = 2.9
  dimension "d268" = 2.9
  constraint concentric A1 A10
  constraint concentric A2 A11
  constraint concentric A0 A12
  measures "d266" diameter of A10
  measures "d267" diameter of A11
  measures "d268" diameter of A12
extrude "Extrude39" cut sketch "Sketch23" against normal blind 5 contours A10 | A11 | A12 picked at (-25.53814, -15.142465) picked at (25.698647, -15.662815) picked at (-0.399349, 29.727729)
extrude "Extrude40" add 2 faces at (-19.283471, 0, 13.127844) (21.482761, 0, 12.949624) along direction (0, -1, 0) blind 4
extrude "Extrude43" add 3 faces at (5.333333, -1.333333, 39.796081) (-5.333333, -1.333333, 39.796081) (0, 2.666667, 39.796081) along direction (0, 0, 1) blind 4
extrude "Extrude44" add 2 faces at (-15.974211, 0, 37.942103) (15.974211, 0, 37.478071) along direction (0, -1, 0) blind 4
sketch "Sketch26" plane through (-16, 0, 0) normal (-1, 0, 0) x (0, -1, 0)
  line L0 (4, 14.796081) -> (4, 43.796081)
  line L1 (4, 43.796081) -> (-4, 43.796081)
  line L2 (-4, 43.796081) -> (-4, 14.796081)
  line L3 (-4, 14.796081) -> (4, 14.796081)
  line L4 (0, 43.796081) -> (0, 36.296081)
  line L5 (0, 36.296081) -> (0, 22.796081)
  circle A0 centre (0, 36.296081) radius 1.425
  circle A1 centre (0, 22.796081) radius 1.425
  dimension "d293" = 7.5
  dimension "d294" = 13.5
  dimension "d295" = 2.85
  dimension "d296" = 2.85
  constraint perpendicular L1 L4
  constraint parallel L4 L5
  measures "d295" diameter of A0
  measures "d296" diameter of A1
sketch "Sketch27" plane through (16, 0, 0) normal (1, 0, 0) x (0, 1, 0)
  line L0 (-4, 14.796081) -> (4, 14.796081)
  line L1 (4, 14.796081) -> (4, 43.796081)
  line L2 (4, 43.796081) -> (-4, 43.796081)
  line L3 (-4, 43.796081) -> (-4, 14.796081)
  line L4 (0, 43.796081) -> (0, 36.296081)
  line L5 (0, 36.296081) -> (0, 22.796081)
  circle A0 centre (0, 36.296081) radius 1.425
  circle A1 centre (0, 22.796081) radius 1.425
  dimension "d297" = 7.5
  dimension "d298" = 13.5
  dimension "d299" = 2.85
  dimension "d300" = 2.85
  constraint perpendicular L2 L4
  constraint perpendicular L2 L5
  measures "d299" diameter of A0
  measures "d300" diameter of A1
extrude "Extrude45" cut sketch "Sketch27" against normal blind 5 contours L4 L5 A0 | L4 L5 A0 | A1 picked at (0.945165, 36.228481) picked at (-0.070795, 35.351386) picked at (-0.235794, 23.168486)
extrude "Extrude46" cut sketch "Sketch26" against normal blind 5 contours L4 L5 A0 | L4 L5 A0 | A1 picked at (0.945165, 36.228481) picked at (-0.070795, 35.351386) picked at (0.218055, 23.150493)
fillet "Fillet8" radius 5 2 edges at (16, 0, 43.796081) (-16, 0, 43.796081)
fillet "Fillet9" radius 6 2 edges at (32, 0, -22.203919) (-32, 0, -22.203919)
extrude "Extrude47" cut 1 faces at (-2.051955, 10, -6.788293) along direction (0, 1, 0) blind 4
